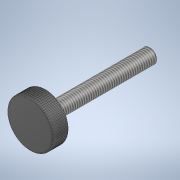
# Autodesk Inventor part: Thumbscrew M5 - Long
Saved by Autodesk Inventor 2020 (Build 240168000, 168)
## iProperties
Created: 2020-02-14
Part Number: Thumbscrew M5 - Long
Material: ABS Plastic
Document SubType Name: Modeling
Designer: Ishaan
Density: 1.06 g/cm^3
Appearance: Smooth - Black
Author: Ishaan
Autodesk Inventor part; units mm, degrees
ref_plane "YZ Plane" through (0, 0, 0) normal (1, 0, 0) x (0, 1, 0)
ref_plane "XZ Plane" through (0, 0, 0) normal (0, 1, 0) x (-1, 0, 0)
ref_plane "XY Plane" through (0, 0, 0) normal (0, 0, 1) x (1, 0, 0)
sketch "Sketch1" plane through (0, 0, 0) normal (0, 0, 1) x (1, 0, 0)
  circle A0 centre (0, 0) radius 8
  dimension "d0" = 16
  constraints: 1 centre point, 1 coincident
  measures "d0" diameter of A0
extrude "Extrusion1" add sketch "Sketch1" along normal blind 6.5
sketch "Sketch2" plane through (0, 0, 0) normal (0, 0, -1) x (-1, 0, 0)
  circle A0 centre (0, 0) radius 2.5
  dimension "d3" = 5
  constraints: 1 centre point, 1 coincident
  measures "d3" diameter of A0
extrude "Extrusion2" add sketch "Sketch2" along normal blind 35
sketch "Sketch3" plane through (0, 0, 0) normal (0, 0, -1) x (-1, 0, 0)
  circle A0 centre (0, 0) radius 2.5 projected
  circle A1 centre (0, 0) radius 8 projected
  circle A2 centre (0, 0) radius 6
  dimension "d7" = 12
  constraints: 1 centre point
  measures "d7" diameter of A2
extrude "Extrusion3" cut sketch "Sketch3" against normal blind 1 contours A1
chamfer "Chamfer1" distance 0.25 angle 45 1 edges at (2.5, 0, -35)
fillet "Fillet1" radius 0.5 2 edges at (-8, 0, 1) (-8, 0, 6.5)
fillet "Fillet2" radius 0.25 2 edges at (6, 0, 1) (6, 0, 0)
thread "Thread1" size "M5x0.8" class "6g" standard "ANSI Metric M Profile" full length
sketch "Sketch4" plane through (0, 0, 6.5) normal (0, 0, 1) x (1, 0, 0)
  circle A0 centre (0, 0) radius 7.5 projected
  circle A1 centre (0, 0) radius 7.5 projected
  circle A2 centre (0, 0) radius 7.5 projected
  circle A3 centre (0, 0) radius 7.5 projected
  circle A4 centre (0, 0) radius 8 projected
  line L0 (8, -0.1875) -> (7.75, -0.1875)
  line L1 (7.75, -0.1875) -> (7.75, 0.1875)
  line L2 (7.75, 0.1875) -> (8, 0.1875)
  line L3 (8, 0.1875) -> (8, -0.1875)
  line L4 (8, -0.1875) -> (7.75, 0.1875) construction
  line L5 (7.75, -0.1875) -> (8, 0.1875) construction
  point P0 (7.875, 0)
  point P1 (7.875, 0)
  dimension "d17" = 0.375
  dimension "d18" = 0.25
  constraints: 12 end point, 3 midpoint, 2 parallel, 1 horizontal, 1 horizontal alignment, 1 perpendicular, 1 tangent
  measures "d17" distance between parallel lines of L0 L2
  measures "d18" distance between parallel lines of L1 L3
extrude "Extrusion4" cut sketch "Sketch4" against normal through all contours A4 L0 L1 L2 | L3 L0 A4 | A4 L2 L3 picked at (7.8333, 0)
pattern_circular "Circular Pattern1" count 75 over 360 about axis through (0, 0, -10) along (0, 0, 1) of "Extrusion4"
body "Solid1"
